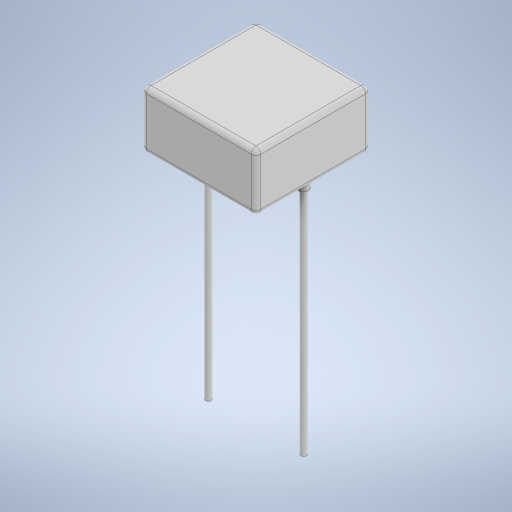
# Autodesk Inventor part: Деталь1
Saved by Autodesk Inventor 2024 (Build 280153000, 153)
## iProperties
Created: 2023-12-19
Part Number: Деталь1
Material: Типовые
Document SubType Name: Sheet Metal
Designer: XoTTaBbl4
Density: 1 g/cm^3
Sheet Metal Rule: По умолчанию_мм
Appearance: По умолчанию
Author: XoTTaBbl4
Autodesk Inventor part; units mm, degrees
ref_plane "YZ Plane" through (0, 0, 0) normal (1, 0, 0) x (0, 1, 0)
ref_plane "XZ Plane" through (0, 0, 0) normal (0, 1, 0) x (-1, 0, 0)
ref_plane "XY Plane" through (0, 0, 0) normal (0, 0, 1) x (1, 0, 0)
sketch "Эскиз7" plane through (0, 0, 0) normal (0, 1, 0) x (-1, 0, 0)
  line L0 (-6, 6) -> (6, 6)
  line L1 (6, 6) -> (6, -6)
  line L2 (6, -6) -> (-6, -6)
  line L3 (-6, -6) -> (-6, 6)
  line L4 (-6, 6) -> (6, -6) construction
  line L5 (6, 6) -> (-6, -6) construction
  point P0 (0, 0)
  dimension "d12" = 12
  dimension "d13" = 12
  constraints: 12 end point, 2 midpoint, 2 parallel, 1 horizontal, 1 perpendicular
  measures "d12" distance of L1.end L2.end
  measures "d13" distance of L0.end L1.end
extrude "Выдавливание2" add sketch "Эскиз7" along normal blind 6
fillet "Сопряжение1" radius 0.5 1 edges at (6, 6, 0)
fillet "Сопряжение2" radius 0.5 13 edges at (6, 2.75, 6) (5.8536, 5.8536, 6) (-0.25, 6, 6) (-6, 0, 0) (6, 0, 0) (5.8536, 5.8536, -6) (-0.25, 6, -6) (6, 2.75, -6) (-6, 3, -6) (-6, 6, 0) (0, 0, 6) (-6, 3, 6) (0, 0, -6)
sketch "Эскиз8" plane through (0, 0, 0) normal (0, -1, 0) x (1, 0, 0)
  line L0 (0, 0) -> (-5, 0)
  line L1 (0, 0) -> (5, 0)
  circle A0 centre (-5, 0) radius 0.5
  circle A1 centre (5, 0) radius 0.5
  line L2 (5.5, -5.5) -> (5.5, 5.5) projected
  dimension "d18" = 5
  dimension "d19" = 5
  constraints: 4 end point, 2 centre point, 2 coincident, 2 horizontal, 1 tangent
  measures "d18" distance of L0.start L0.end
  measures "d19" distance of L0.start L1.end
extrude "Выдавливание3" add sketch "Эскиз8" along normal blind 1
fillet "Сопряжение3" radius 0.2 1 edges at (-5.5, -1, 0)
fillet "Сопряжение4" radius 0.2 1 edges at (4.5, -1, 0)
sketch "Эскиз10" plane through (-5, -1, 0) normal (0, -1, 0) x (1, 0, 0)
  circle A0 centre (0, 0) radius 0.3
  point P0 (5, 0)
  constraints: 1 centre point
extrude "Выдавливание4" add sketch "Эскиз10" along normal blind 24
sketch "Эскиз11" plane through (5, -1, 0) normal (0, -1, 0) x (1, 0, 0)
  circle A0 centre (0, 0) radius 0.3 projected
  circle A1 centre (0, 0) radius 0.3
  point P0 (-5, 0)
  constraints: 1 centre point, 1 coincident
extrude "Выдавливание5" add sketch "Эскиз11" along normal blind 24
equation "\"Радиус_гибки\" = Толщина"
equation "\"Ширина_просечки\" = Толщина"
equation "\"Глубина_просечки\" = 0.5 * Толщина"
equation "\"Размер_просечки\" = 4 * Толщина"
equation "\"Мин_остаток\" = 2 * Толщина"
equation "\"Радиус_перехода\" = Радиус_гибки"
equation "\"Радиус_Якоби\" = Радиус_гибки"
equation "\"Размер_зазора\" = Толщина"
equation "\"Толщина\" = 0.5"
